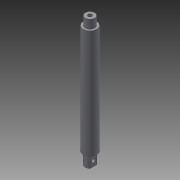
# Autodesk Inventor part: Small_piston
Saved by Autodesk Inventor 2015 (Build 190159000, 159)
## iProperties
Created: 2017-02-22
Part Number: Small_piston
Material: Aluminum 6061-AHC
Document SubType Name: Modeling
Designer: Guy
Density: 2.7 g/cm^3
Appearance: Aluminum - Dark
Mass: 65.5669 g
Surface Area: 94.8654 cm^2
Volume: 24.284 cm^3
Author: Guy
Autodesk Inventor part; units mm, degrees
ref_plane "YZ Plane" through (0, 0, 0) normal (1, 0, 0) x (0, 1, 0)
ref_plane "XZ Plane" through (0, 0, 0) normal (0, 1, 0) x (-1, 0, 0)
ref_plane "XY Plane" through (0, 0, 0) normal (0, 0, 1) x (1, 0, 0)
sketch "Sketch1" plane through (0, 0, 0) normal (0, 0, 1) x (1, 0, 0)
  circle A0 centre (0, 0) radius 7.875
  dimension "d0" = 15.75
  constraints: 1 centre point, 1 coincident
  measures "d0" diameter of A0
extrude "Extrusion1" add sketch "Sketch1" along normal blind 126
sketch "Sketch2" plane through (0, 0, 126) normal (0, 0, 1) x (1, 0, 0)
  circle A0 centre (0, 0) radius 5.5
  dimension "d3" = 11
  constraints: 1 centre point, 1 coincident
  measures "d3" diameter of A0
extrude "Extrusion2" add sketch "Sketch2" along normal blind 10
sketch "Sketch3" plane through (0, 0, 0) normal (0, 0, -1) x (-1, 0, 0)
  circle A0 centre (0, 0) radius 5.5
  dimension "d6" = 11
  constraints: 1 centre point, 1 coincident
  measures "d6" diameter of A0
extrude "Extrusion3" add sketch "Sketch3" along normal blind 14
sketch "Sketch4" plane through (0, 0, -14) normal (0, 0, -1) x (-1, 0, 0)
  line L0 (4, 13.3221) -> (11.8644, 13.3221)
  line L1 (11.8644, 13.3221) -> (11.8644, -10.8813)
  line L2 (11.8644, -10.8813) -> (4, -10.8813)
  line L3 (4, -10.8813) -> (4, 13.3221)
  line L4 (-11.0508, 13.3221) -> (-4, 13.3221)
  line L5 (-4, 13.3221) -> (-4, -10.8813)
  line L6 (-4, -10.8813) -> (-11.0508, -10.8813)
  line L7 (-11.0508, -10.8813) -> (-11.0508, 13.3221)
  point P0 (0, 0)
  dimension "d9" = 8
  dimension "d10" = 4
  constraints: 16 end point, 5 parallel, 2 collinear, 2 horizontal, 2 perpendicular
  measures "d9" distance between parallel lines of L5 L3
  measures "d10" distance from line of point (0, 0) L3
extrude "Extrusion4" cut sketch "Sketch4" against normal up to surface (14 mm away)
sketch "Sketch5" plane through (4, -3.7749, -14) normal (1, 0, 0) x (0, 0, -1)
  circle A0 centre (-6, 3.7748) radius 2
  line L0 (0, 7.5498) -> (0, 0) projected
  line L1 (-14, 7.5498) -> (0, 7.5498) projected
  point P0 (-14, 3.7749)
  dimension "d13" = 4
  dimension "d14" = 6
  dimension "d15" = 3.775
  constraints: 1 centre point
  measures "d13" diameter of A0
  measures "d14" distance from line of A0.centre L0
  measures "d15" distance from line of A0.centre L1
extrude "Extrusion5" cut sketch "Sketch5" against normal up to next
sketch "Sketch7" plane through (0, 0, 136) normal (0, 0, 1) x (1, 0, 0)
  circle A0 centre (0, 0) radius 2.25
  dimension "d21" = 4.5
  constraints: 1 centre point, 1 coincident
  measures "d21" diameter of A0
extrude "Extrusion7" cut sketch "Sketch7" against normal blind 140
body "Solid1"
